Autodesk Inventor part; units mm, degrees
(part 4 of 6)
sketch "S09_267p4" plane through (0, 0, 0) normal (0, 0, 1) x (1, 0, 0)
  spline S0 degree 4 poles (184.2102, -33.211) (184.1723, -33.1957) (183.9876, -33.1195) (183.6772, -32.9928) (183.1534, -32.7788) (182.6023, -32.5533) (181.925, -32.2782) (181.1275, -31.9535) (180.2077, -31.5815) (179.1682, -31.1613) (178.009, -30.6956) (176.7313, -30.1834) (175.3365, -29.6271) (173.8252, -29.0272) (172.1997, -28.3847) (170.46, -27.7017) (168.6088, -26.9787) (166.6473, -26.2177) (164.5772, -25.419) (162.4002, -24.5854) (160.1184, -23.7178) (157.7339, -22.8179) (155.2484, -21.8869) (152.665, -20.9269) (149.9848, -19.9394) (147.2115, -18.9267) (144.3465, -17.889) (141.3934, -16.8298) (138.3539, -15.7493) (135.2318, -14.6509) (132.029, -13.5347) (128.7493, -12.404) (125.3952, -11.2596) (121.9703, -10.104) (118.4772, -8.9384) (114.92, -7.765) (111.3009, -6.5858) (107.6244, -5.4023) (103.8935, -4.2167) (100.1117, -3.0305) (96.2827, -1.8459) (92.4099, -0.6646) (88.4973, 0.5118) (84.5488, 1.6811) (80.5675, 2.8412) (76.5582, 3.9907) (72.5236, 5.1283) (68.4687, 6.2504) (64.3965, 7.3573) (60.3118, 8.4456) (56.2177, 9.5148) (52.1191, 10.5622) (48.0189, 11.5858) (43.9221, 12.5858) (39.832, 13.5582) (35.7496, 14.504) (31.6853, 15.4187) (27.6208, 16.3072) (23.5666, 17.1536) (19.5384, 17.959) (15.537, 18.7209) (11.5694, 19.4378) (7.6397, 20.1105) (3.7522, 20.7356) (-0.0895, 21.3157) (-3.8804, 21.8471) (-7.6174, 22.3317) (-11.2958, 22.7677) (-14.9121, 23.1565) (-18.462, 23.4964) (-21.9422, 23.7889) (-25.3485, 24.0333) (-28.6772, 24.2307) (-31.9251, 24.3805) (-35.0882, 24.4845) (-38.1632, 24.5425) (-41.1473, 24.5559) (-44.0366, 24.5247) (-46.8284, 24.4513) (-49.5195, 24.3353) (-52.1073, 24.178) (-54.5888, 23.9818) (-56.9615, 23.7464) (-59.2228, 23.4736) (-61.3709, 23.1653) (-63.4029, 22.8217) (-65.3171, 22.445) (-67.1116, 22.0362) (-68.7849, 21.5965) (-70.3349, 21.1268) (-71.761, 20.629) (-73.0614, 20.104) (-74.2351, 19.5519) (-75.2824, 18.9753) (-76.201, 18.3724) (-76.9918, 17.7451) (-77.6536, 17.0931) (-78.1852, 16.4152) (-78.5837, 15.7115) (-78.8483, 14.9847) (-78.9751, 14.2355) (-78.9672, 13.4757) (-78.8207, 12.7166) (-78.5387, 11.9594) (-78.1238, 11.2064) (-77.5783, 10.4572) (-76.904, 9.7121) (-76.102, 8.9696) (-75.1736, 8.2296) (-74.1195, 7.4923) (-72.9408, 6.7577) (-71.6387, 6.0264) (-70.2144, 5.2983) (-68.6696, 4.5743) (-67.0057, 3.8541) (-65.2248, 3.1392) (-63.3284, 2.4284) (-61.3186, 1.7241) (-59.1974, 1.0249) (-56.9673, 0.3318) (-54.63, -0.3546) (-52.1885, -1.0338) (-49.6448, -1.7073) (-47.0016, -2.3723) (-44.2618, -3.0312) (-41.4273, -3.6822) (-38.5019, -4.3262) (-35.488, -4.9635) (-32.3885, -5.5926) (-29.2065, -6.2163) (-25.9449, -6.8317) (-22.6074, -7.4421) (-19.1967, -8.0454) (-15.716, -8.6434) (-12.1695, -9.2365) (-8.5591, -9.8239) (-4.89, -10.4076) (-1.1645, -10.9871) (2.6133, -11.5629) (6.44, -12.1363) (10.3116, -12.7077) (14.2249, -13.2764) (18.1779, -13.8455) (22.1649, -14.4118) (26.1914, -14.983) (30.265, -15.5476) (34.3574, -16.1047) (38.4734, -16.6535) (42.6033, -17.1948) (46.7445, -17.7289) (50.8923, -18.2558) (55.0422, -18.7753) (59.1903, -19.2884) (63.3327, -19.7938) (67.465, -20.2937) (71.5831, -20.7858) (75.6829, -21.2723) (79.7601, -21.7518) (83.8113, -22.224) (87.8314, -22.6905) (91.817, -23.1497) (95.7643, -23.6014) (99.6691, -24.0469) (103.527, -24.4841) (107.3352, -24.9145) (111.0889, -25.3368) (114.7848, -25.7508) (118.4191, -26.1563) (121.9885, -26.5536) (125.4884, -26.9419) (128.9164, -27.3206) (132.2686, -27.6896) (135.5413, -28.0495) (138.7315, -28.398) (141.8361, -28.7371) (144.8517, -29.0645) (147.7753, -29.3818) (150.604, -29.6867) (153.3349, -29.9808) (155.9649, -30.2626) (158.4918, -30.5326) (160.9125, -30.7897) (163.2249, -31.0354) (165.4264, -31.2674) (167.5147, -31.4874) (169.4878, -31.6945) (171.3435, -31.8878) (173.0798, -32.0687) (174.6952, -32.2366) (176.1875, -32.3905) (177.5553, -32.5317) (178.7975, -32.659) (179.912, -32.7736) (180.8985, -32.8742) (181.755, -32.9616) (182.4819, -33.0358) (183.0744, -33.0955) (183.6373, -33.1534) (183.9708, -33.1866) (184.1695, -33.2068) (184.2102, -33.211) knots 0 0 0 0 0 0.003306 0.005253 0.00752 0.010062 0.01285 0.015861 0.019079 0.022488 0.026078 0.029837 0.033757 0.037828 0.042045 0.046398 0.050884 0.055494 0.060224 0.065069 0.070023 0.075082 0.080241 0.085495 0.090841 0.096274 0.101791 0.107386 0.113057 0.118799 0.124609 0.130484 0.136419 0.142412 0.148458 0.154554 0.160697 0.166884 0.17311 0.179374 0.185671 0.191998 0.198352 0.20473 0.211128 0.217543 0.223972 0.230412 0.23686 0.243312 0.249765 0.256217 0.262663 0.2691 0.275526 0.281941 0.288345 0.294734 0.301105 0.307451 0.313767 0.320049 0.326294 0.332498 0.338659 0.344773 0.350837 0.356848 0.362801 0.368695 0.374525 0.380288 0.38598 0.391599 0.39714 0.4026 0.407976 0.413263 0.418458 0.423557 0.428556 0.433452 0.438241 0.442917 0.447478 0.451919 0.456236 0.460425 0.464482 0.468403 0.472185 0.475825 0.479322 0.482675 0.485889 0.48897 0.49193 0.494788 0.497572 0.50031 0.503032 0.505769 0.508552 0.511409 0.514365 0.517441 0.520647 0.523991 0.527474 0.531098 0.534861 0.538758 0.542789 0.546947 0.551231 0.555634 0.560154 0.564786 0.569527 0.574371 0.579315 0.584356 0.58949 0.594712 0.60002 0.605409 0.610877 0.61642 0.622034 0.627716 0.633463 0.639271 0.645138 0.651061 0.657035 0.663059 0.669128 0.675241 0.681393 0.687582 0.693804 0.700057 0.706341 0.712655 0.718998 0.725365 0.731751 0.738149 0.744556 0.750969 0.757385 0.7638 0.770211 0.776616 0.783011 0.789393 0.795759 0.802106 0.808429 0.814727 0.820996 0.827232 0.833433 0.839595 0.845714 0.851788 0.857813 0.863785 0.869702 0.875558 0.881352 0.887078 0.892735 0.898316 0.90382 0.909242 0.914577 0.919822 0.924972 0.930023 0.93497 0.939808 0.944533 0.949139 0.95362 0.95797 0.962183 0.966252 0.970169 0.973927 0.977515 0.980924 0.984141 0.987151 0.989939 0.99248 0.994747 0.996694 1 1 1 1 1
  circle A0 centre (0, 0) radius 5.15
  line L0 (-32.24, 4.9) -> (-22.04, 4.9)
  line L1 (-22.04, 4.9) -> (-22.04, 9.1)
  line L2 (-22.04, 9.1) -> (-32.24, 9.1)
  line L3 (-32.24, 9.1) -> (-32.24, 4.9)
  line L4 (-32.24, 4.9) -> (-22.04, 9.1) construction
  line L5 (-22.04, 4.9) -> (-32.24, 9.1) construction
  line L6 (-58.58, 15.1) -> (-48.38, 15.1)
  line L7 (-48.38, 15.1) -> (-48.38, 10.9)
  line L8 (-48.38, 10.9) -> (-58.58, 10.9)
  line L9 (-58.58, 10.9) -> (-58.58, 15.1)
  line L10 (-58.58, 15.1) -> (-48.38, 10.9) construction
  line L11 (-48.38, 15.1) -> (-58.58, 10.9) construction
  line L12 (44.9, -2.9) -> (55.1, -2.9)
  line L13 (55.1, -2.9) -> (55.1, -7.1)
  line L14 (55.1, -7.1) -> (44.9, -7.1)
  line L15 (44.9, -7.1) -> (44.9, -2.9)
  line L16 (44.9, -2.9) -> (55.1, -7.1) construction
  line L17 (55.1, -2.9) -> (44.9, -7.1) construction
  line L18 (97.6, -12.9) -> (87.4, -12.9)
  line L19 (87.4, -12.9) -> (87.4, -17.1)
  line L20 (87.4, -17.1) -> (97.6, -17.1)
  line L21 (97.6, -17.1) -> (97.6, -12.9)
  line L22 (97.6, -12.9) -> (87.4, -17.1) construction
  line L23 (87.4, -12.9) -> (97.6, -17.1) construction
  point P0 (183.963, -33.1097)
  point P1 (183.654, -32.9833)
  point P2 (183.222, -32.8068)
  point P3 (182.6673, -32.5802)
  point P4 (181.9901, -32.3046)
  point P5 (181.1912, -31.9798)
  point P6 (180.2709, -31.6072)
  point P7 (179.2305, -31.187)
  point P8 (178.0707, -30.7206)
  point P9 (176.7923, -30.2083)
  point P10 (175.3966, -29.6516)
  point P11 (173.8846, -29.0513)
  point P12 (172.258, -28.4086)
  point P13 (170.5176, -27.7251)
  point P14 (168.6653, -27.0018)
  point P15 (166.7028, -26.2401)
  point P16 (164.6316, -25.4412)
  point P17 (162.4535, -24.607)
  point P18 (160.1705, -23.7389)
  point P19 (157.7848, -22.8384)
  point P20 (155.2981, -21.907)
  point P21 (152.7131, -20.9465)
  point P22 (150.0318, -19.9585)
  point P23 (147.2569, -18.9449)
  point P24 (144.3905, -17.907)
  point P25 (141.4358, -16.8469)
  point P26 (138.3948, -15.7661)
  point P27 (135.2711, -14.6669)
  point P28 (132.0668, -13.5503)
  point P29 (128.7852, -12.4188)
  point P30 (125.4295, -11.2739)
  point P31 (122.0028, -10.1176)
  point P32 (118.508, -8.9515)
  point P33 (114.9488, -7.7775)
  point P34 (111.328, -6.5976)
  point P35 (107.6495, -5.4135)
  point P36 (103.9167, -4.2273)
  point P37 (100.133, -3.0405)
  point P38 (96.302, -1.8553)
  point P39 (92.4272, -0.6734)
  point P40 (88.5126, 0.5035)
  point P41 (84.562, 1.6733)
  point P42 (80.5788, 2.8341)
  point P43 (76.5673, 3.9842)
  point P44 (72.5307, 5.1219)
  point P45 (68.4735, 6.2449)
  point P46 (64.3994, 7.352)
  point P47 (60.3125, 8.4409)
  point P48 (56.2163, 9.5104)
  point P49 (52.1154, 10.5581)
  point P50 (48.0133, 11.5824)
  point P51 (43.9144, 12.5822)
  point P52 (39.8223, 13.5553)
  point P53 (35.7415, 14.5002)
  point P54 (31.6757, 15.4153)
  point P55 (27.6092, 16.3014)
  point P56 (23.5509, 17.1494)
  point P57 (19.518, 17.955)
  point P58 (15.5145, 18.717)
  point P59 (11.5448, 19.4343)
  point P60 (7.6131, 20.1065)
  point P61 (3.7236, 20.7322)
  point P62 (-0.1199, 21.3115)
  point P63 (-3.9127, 21.8432)
  point P64 (-7.6514, 22.3273)
  point P65 (-11.3316, 22.7634)
  point P66 (-14.9496, 23.1516)
  point P67 (-18.5013, 23.4914)
  point P68 (-21.9831, 23.7833)
  point P69 (-25.3909, 24.0273)
  point P70 (-28.7211, 24.224)
  point P71 (-31.9705, 24.3734)
  point P72 (-35.135, 24.4766)
  point P73 (-38.2113, 24.534)
  point P74 (-41.1965, 24.5464)
  point P75 (-44.087, 24.5146)
  point P76 (-46.8798, 24.4399)
  point P77 (-49.5718, 24.3229)
  point P78 (-52.1604, 24.1646)
  point P79 (-54.6425, 23.9668)
  point P80 (-57.0157, 23.7301)
  point P81 (-59.2774, 23.4558)
  point P82 (-61.4255, 23.1456)
  point P83 (-63.4574, 22.8003)
  point P84 (-65.3711, 22.4215)
  point P85 (-67.1649, 22.0105)
  point P86 (-68.8368, 21.5683)
  point P87 (-70.3851, 21.0961)
  point P88 (-71.8087, 20.5955)
  point P89 (-73.1057, 20.0675)
  point P90 (-74.2751, 19.5129)
  point P91 (-75.3162, 18.9333)
  point P92 (-76.2275, 18.3289)
  point P93 (-77.0088, 17.7011)
  point P94 (-77.6594, 17.0508)
  point P95 (-78.1787, 16.3782)
  point P96 (-78.5664, 15.684)
  point P97 (-78.8227, 14.9689)
  point P98 (-78.9472, 14.2333)
  point P99 (-78.9396, 13.4872)
  point P100 (-78.7992, 12.7407)
  point P101 (-78.5268, 11.9944)
  point P102 (-78.1227, 11.2483)
  point P103 (-77.5877, 10.5027)
  point P104 (-76.9225, 9.7584)
  point P105 (-76.128, 9.0152)
  point P106 (-75.2056, 8.2737)
  point P107 (-74.1561, 7.5343)
  point P108 (-72.981, 6.7974)
  point P109 (-71.6816, 6.0638)
  point P110 (-70.2593, 5.3335)
  point P111 (-68.716, 4.6072)
  point P112 (-67.0531, 3.8852)
  point P113 (-65.2728, 3.168)
  point P114 (-63.3767, 2.4558)
  point P115 (-61.3671, 1.7495)
  point P116 (-59.2458, 1.0489)
  point P117 (-57.0153, 0.3544)
  point P118 (-54.6775, -0.3333)
  point P119 (-52.2353, -1.0141)
  point P120 (-49.6909, -1.6883)
  point P121 (-47.0469, -2.3549)
  point P122 (-44.3061, -3.0145)
  point P123 (-41.4707, -3.6667)
  point P124 (-38.5441, -4.3117)
  point P125 (-35.529, -4.9496)
  point P126 (-32.4283, -5.5801)
  point P127 (-29.245, -6.204)
  point P128 (-25.982, -6.8208)
  point P129 (-22.643, -7.4315)
  point P130 (-19.2309, -8.0358)
  point P131 (-15.7487, -8.6345)
  point P132 (-12.2004, -9.228)
  point P133 (-8.5887, -9.8164)
  point P134 (-4.9177, -10.4005)
  point P135 (-1.1906, -10.9807)
  point P136 (2.589, -11.5572)
  point P137 (6.4174, -12.1311)
  point P138 (10.2909, -12.7028)
  point P139 (14.2057, -13.2725)
  point P140 (18.1582, -13.8411)
  point P141 (22.1445, -14.4087)
  point P142 (26.1741, -14.9779)
  point P143 (30.25, -15.5434)
  point P144 (34.3485, -16.1011)
  point P145 (38.4663, -16.6506)
  point P146 (42.5987, -17.1924)
  point P147 (46.7418, -17.7269)
  point P148 (50.8917, -18.2542)
  point P149 (55.0437, -18.7742)
  point P150 (59.1939, -19.2874)
  point P151 (63.3384, -19.7936)
  point P152 (67.4728, -20.2934)
  point P153 (71.5931, -20.7862)
  point P154 (75.6949, -21.2728)
  point P155 (79.7742, -21.7526)
  point P156 (83.8274, -22.2254)
  point P157 (87.8497, -22.6919)
  point P158 (91.8373, -23.1514)
  point P159 (95.7866, -23.6037)
  point P160 (99.6934, -24.0491)
  point P161 (103.5535, -24.4869)
  point P162 (107.3635, -24.9173)
  point P163 (111.1193, -25.3398)
  point P164 (114.817, -25.754)
  point P165 (118.4533, -26.1599)
  point P166 (122.0244, -26.5573)
  point P167 (125.5263, -26.9458)
  point P168 (128.956, -27.3247)
  point P169 (132.31, -27.6941)
  point P170 (135.5845, -28.0538)
  point P171 (138.7764, -28.4029)
  point P172 (141.8826, -28.7417)
  point P173 (144.8998, -29.0697)
  point P174 (147.8249, -29.3868)
  point P175 (150.6552, -29.6922)
  point P176 (153.3875, -29.9861)
  point P177 (156.019, -30.2682)
  point P178 (158.5472, -30.5382)
  point P179 (160.9692, -30.7958)
  point P180 (163.2829, -31.0412)
  point P181 (165.4856, -31.2736)
  point P182 (167.5751, -31.4936)
  point P183 (169.5492, -31.7006)
  point P184 (171.406, -31.8943)
  point P185 (173.1433, -32.0752)
  point P186 (174.7596, -32.243)
  point P187 (176.2528, -32.3973)
  point P188 (177.6215, -32.5383)
  point P189 (178.8644, -32.666)
  point P190 (179.9798, -32.7804)
  point P191 (180.967, -32.8812)
  point P192 (181.8247, -32.9687)
  point P193 (182.5518, -33.0427)
  point P194 (183.1482, -33.1032)
  point P195 (183.6124, -33.1505)
  point P196 (183.9444, -33.184)
  point P197 (184.1437, -33.2042)
  point P198 (-27.14, 7)
  point P199 (-53.48, 13)
  dimension "d16" = 10.3
  dimension "d17" = 80.22
  dimension "d88" = 10.2
  dimension "d89" = 4.2
  dimension "d91" = 10.2
  dimension "d92" = 4.2
  dimension "d155" = 27.14
  dimension "d156" = 7
  dimension "d157" = 53.48
  dimension "d158" = 13
  dimension "d251" = 10.2
  dimension "d252" = 4.2
  dimension "d253" = 50
  dimension "d254" = 5
  dimension "d255" = 10.2
  dimension "d256" = 4.2
  dimension "d257" = 92.5
  dimension "d258" = 15
  constraints: 48 end point, 8 midpoint, 8 parallel, 4 horizontal, 4 perpendicular, 1 centre point, 201 other
  measures "d16" diameter of A0
  measures "d17" distance of A0.centre point (-78.947, 14.233)
  measures "d88" distance of L2.end L1.end
  measures "d89" distance of L1.end L0.end
  measures "d91" distance of L7.end L8.end
  measures "d92" distance of L6.end L7.end
  measures "d155" horizontal distance of point (-27.14, 7) point (0, 0)
  measures "d156" vertical distance of point (0, 0) point (-27.14, 7)
  measures "d157" horizontal distance of point (0, 0) point (-53.48, 13)
  measures "d158" vertical distance of point (0, 0) point (-53.48, 13)
  measures "d251" distance of L13.end L14.end
  measures "d252" distance of L12.end L13.end
  measures "d253" horizontal distance of point (50, -5) point (0, 0)
  measures "d254" vertical distance of point (0, 0) point (50, -5)
  measures "d255" distance of L20.end L19.end
  measures "d256" distance of L19.end L18.end
  measures "d257" horizontal distance of point (92.5, -15) point (0, 0)
  measures "d258" vertical distance of point (0, 0) point (92.5, -15)
sketch "S10_259p0" plane through (0, 0, 0) normal (0, 0, 1) x (1, 0, 0)
  spline S0 degree 4 poles (176.9199, -39.6111) (176.8839, -39.5948) (176.7082, -39.5135) (176.413, -39.3784) (175.9147, -39.15) (175.3906, -38.9094) (174.7463, -38.6158) (173.9877, -38.2692) (173.1127, -37.8719) (172.1237, -37.4231) (171.0208, -36.9253) (169.8051, -36.3778) (168.4779, -35.7829) (167.0397, -35.1411) (165.4927, -34.4534) (163.8368, -33.7219) (162.0747, -32.9471) (160.2073, -32.1311) (158.2364, -31.2742) (156.1634, -30.3792) (153.9905, -29.447) (151.7194, -28.4794) (149.3519, -27.4777) (146.8907, -26.4439) (144.3371, -25.3795) (141.6943, -24.2869) (138.9638, -23.1666) (136.149, -22.0217) (133.2513, -20.8528) (130.2746, -19.6633) (127.2204, -18.4532) (124.0923, -17.226) (120.8929, -15.9824) (117.6253, -14.7252) (114.2922, -13.4555) (110.8974, -12.1757) (107.4428, -10.8877) (103.9329, -9.5932) (100.3705, -8.2946) (96.7588, -6.9933) (93.1014, -5.6916) (89.4015, -4.3913) (85.6629, -3.0942) (81.8892, -1.8024) (78.0833, -0.5183) (74.25, 0.7568) (70.3918, 2.0213) (66.5132, 3.2717) (62.6173, 4.508) (58.7085, 5.7269) (54.7898, 6.9276) (50.8659, 8.1075) (46.9396, 9.2643) (43.0155, 10.3982) (39.0968, 11.5052) (35.1845, 12.5861) (31.2884, 13.636) (27.3911, 14.6608) (23.502, 15.6444) (19.6365, 16.5871) (15.7951, 17.4867) (11.9846, 18.3415) (8.2089, 19.1518) (4.4721, 19.9145) (0.7779, 20.6316) (-2.8691, 21.2996) (-6.4659, 21.9202) (-10.0079, 22.4913) (-13.4917, 23.0143) (-16.9134, 23.4872) (-20.2694, 23.9114) (-23.5559, 24.286) (-26.7691, 24.6121) (-29.9062, 24.8888) (-32.9631, 25.1177) (-35.9365, 25.2986) (-38.8238, 25.4326) (-41.6211, 25.5196) (-44.3259, 25.5618) (-46.9348, 25.5587) (-49.4455, 25.5114) (-51.8549, 25.4222) (-54.1606, 25.2906) (-56.36, 25.1183) (-58.4513, 24.9071) (-60.4316, 24.6571) (-62.2994, 24.3701) (-64.0526, 24.0473) (-65.6897, 23.6896) (-67.2087, 23.298) (-68.609, 22.8741) (-69.8888, 22.4188) (-71.047, 21.932) (-72.0839, 21.4165) (-72.9974, 20.8704) (-73.7881, 20.2954) (-74.4549, 19.6912) (-74.9969, 19.0568) (-75.4111, 18.3919) (-75.6966, 17.6993) (-75.8498, 16.9795) (-75.8728, 16.2439) (-75.7619, 15.5033) (-75.5197, 14.7591) (-75.1488, 14.0135) (-74.6512, 13.2664) (-74.0289, 12.518) (-73.2829, 11.7669) (-72.4145, 11.0132) (-71.4243, 10.2569) (-70.3134, 9.4982) (-69.083, 8.7377) (-67.7341, 7.9753) (-66.2686, 7.212) (-64.6876, 6.4475) (-62.9932, 5.6834) (-61.1867, 4.9187) (-59.2704, 4.1556) (-57.246, 3.3929) (-55.1159, 2.6317) (-52.8819, 1.8726) (-50.5466, 1.1164) (-48.1123, 0.3613) (-45.5814, -0.3893) (-42.9567, -1.1382) (-40.2401, -1.8831) (-37.4352, -2.625) (-34.5443, -3.3639) (-31.5704, -4.0985) (-28.5164, -4.8311) (-25.385, -5.5589) (-22.1799, -6.285) (-18.9037, -7.0072) (-15.5595, -7.7271) (-12.1515, -8.4449) (-8.6814, -9.1598) (-5.1544, -9.8735) (-1.5726, -10.5854) (2.06, -11.2959) (5.74, -12.0059) (9.4635, -12.716) (13.2274, -13.4251) (17.0299, -14.1361) (20.8652, -14.8459) (24.7387, -15.562) (28.658, -16.2736) (32.5957, -16.9787) (36.5567, -17.6767) (40.5314, -18.3681) (44.5173, -19.0529) (48.5099, -19.7311) (52.5048, -20.4021) (56.4983, -21.0669) (60.4865, -21.724) (64.4652, -22.3753) (68.4305, -23.0186) (72.3783, -23.6556) (76.3045, -24.2851) (80.2058, -24.9064) (84.0773, -25.5209) (87.9158, -26.1269) (91.7173, -26.7241) (95.4781, -27.3137) (99.1938, -27.8933) (102.8617, -28.4642) (106.4772, -29.0251) (110.037, -29.5757) (113.5376, -30.1156) (116.9757, -30.6447) (120.347, -31.1625) (123.649, -31.668) (126.8781, -32.1611) (130.0306, -32.6421) (133.1038, -33.1088) (136.0945, -33.5628) (138.9995, -34.002) (141.8158, -34.4277) (144.5409, -34.8374) (147.1718, -35.2328) (149.7055, -35.6122) (152.14, -35.9759) (154.4721, -36.323) (156.7, -36.6546) (158.821, -36.9684) (160.833, -37.2659) (162.734, -37.5463) (164.5221, -37.8087) (166.1949, -38.0542) (167.7514, -38.2822) (169.1894, -38.4917) (170.5073, -38.6838) (171.7043, -38.8574) (172.7781, -39.0135) (173.7288, -39.1508) (174.5541, -39.2702) (175.2545, -39.3715) (175.8255, -39.4533) (176.3679, -39.5321) (176.6893, -39.5777) (176.8807, -39.6054) (176.9199, -39.6111) knots 0 0 0 0 0 0.003306 0.005253 0.00752 0.010062 0.01285 0.015861 0.019079 0.022488 0.026078 0.029837 0.033757 0.037828 0.042045 0.046398 0.050884 0.055494 0.060224 0.065069 0.070023 0.075082 0.080241 0.085495 0.090841 0.096274 0.101791 0.107386 0.113057 0.118799 0.124609 0.130484 0.136419 0.142412 0.148458 0.154554 0.160697 0.166884 0.17311 0.179374 0.185671 0.191998 0.198352 0.20473 0.211128 0.217543 0.223972 0.230412 0.23686 0.243312 0.249765 0.256217 0.262663 0.2691 0.275526 0.281941 0.288345 0.294734 0.301105 0.307451 0.313767 0.320049 0.326294 0.332498 0.338659 0.344773 0.350837 0.356848 0.362801 0.368695 0.374525 0.380288 0.38598 0.391599 0.39714 0.4026 0.407976 0.413263 0.418458 0.423557 0.428556 0.433452 0.438241 0.442917 0.447478 0.451919 0.456236 0.460425 0.464482 0.468403 0.472185 0.475825 0.479322 0.482675 0.485889 0.48897 0.49193 0.494788 0.497572 0.50031 0.503032 0.505769 0.508552 0.511409 0.514365 0.517441 0.520647 0.523991 0.527474 0.531098 0.534861 0.538758 0.542789 0.546947 0.551231 0.555634 0.560154 0.564786 0.569527 0.574371 0.579315 0.584356 0.58949 0.594712 0.60002 0.605409 0.610877 0.61642 0.622034 0.627716 0.633463 0.639271 0.645138 0.651061 0.657035 0.663059 0.669128 0.675241 0.681393 0.687582 0.693804 0.700057 0.706341 0.712655 0.718998 0.725365 0.731751 0.738149 0.744556 0.750969 0.757385 0.7638 0.770211 0.776616 0.783011 0.789393 0.795759 0.802106 0.808429 0.814727 0.820996 0.827232 0.833433 0.839595 0.845714 0.851788 0.857813 0.863785 0.869702 0.875558 0.881352 0.887078 0.892735 0.898316 0.90382 0.909242 0.914577 0.919822 0.924972 0.930023 0.93497 0.939808 0.944533 0.949139 0.95362 0.95797 0.962183 0.966252 0.970169 0.973927 0.977515 0.980924 0.984141 0.987151 0.989939 0.99248 0.994747 0.996694 1 1 1 1 1
  circle A0 centre (0, 0) radius 5.15
  line L0 (-48.38, 15.1) -> (-58.58, 15.1)
  line L1 (-58.58, 15.1) -> (-58.58, 10.9)
  line L2 (-58.58, 10.9) -> (-48.38, 10.9)
  line L3 (-48.38, 10.9) -> (-48.38, 15.1)
  line L4 (-48.38, 15.1) -> (-58.58, 10.9) construction
  line L5 (-58.58, 15.1) -> (-48.38, 10.9) construction
  line L6 (-31, 10.1) -> (-20.8, 10.1)
  line L7 (-20.8, 10.1) -> (-20.8, 5.9)
  line L8 (-20.8, 5.9) -> (-31, 5.9)
  line L9 (-31, 5.9) -> (-31, 10.1)
  line L10 (-31, 10.1) -> (-20.8, 5.9) construction
  line L11 (-20.8, 10.1) -> (-31, 5.9) construction
  line L12 (87.4, -12.9) -> (97.6, -12.9)
  line L13 (97.6, -12.9) -> (97.6, -17.1)
  line L14 (97.6, -17.1) -> (87.4, -17.1)
  line L15 (87.4, -17.1) -> (87.4, -12.9)
  line L16 (87.4, -12.9) -> (97.6, -17.1) construction
  line L17 (97.6, -12.9) -> (87.4, -17.1) construction
  line L18 (49.35, -4.9) -> (39.15, -4.9)
  line L19 (39.15, -4.9) -> (39.15, -9.1)
  line L20 (39.15, -9.1) -> (49.35, -9.1)
  line L21 (49.35, -9.1) -> (49.35, -4.9)
  line L22 (49.35, -4.9) -> (39.15, -9.1) construction
  line L23 (39.15, -4.9) -> (49.35, -9.1) construction
  point P0 (0, 0)
  point P1 (176.6848, -39.503)
  point P2 (176.3909, -39.3682)
  point P3 (175.98, -39.1799)
  point P4 (175.4524, -38.9381)
  point P5 (174.8083, -38.6439)
  point P6 (174.0482, -38.2972)
  point P7 (173.1728, -37.8992)
  point P8 (172.183, -37.4504)
  point P9 (171.0795, -36.952)
  point P10 (169.8631, -36.4045)
  point P11 (168.5351, -35.8091)
  point P12 (167.0962, -35.1668)
  point P13 (165.5481, -34.4789)
  point P14 (163.8916, -33.7468)
  point P15 (162.1284, -32.9717)
  point P16 (160.2602, -32.155)
  point P17 (158.2882, -31.2979)
  point P18 (156.2141, -30.4022)
  point P19 (154.0401, -29.4695)
  point P20 (151.7678, -28.5014)
  point P21 (149.3991, -27.4991)
  point P22 (146.9365, -26.4647)
  point P23 (144.3817, -25.3999)
  point P24 (141.7375, -24.3065)
  point P25 (139.0057, -23.1858)
  point P26 (136.1893, -22.04)
  point P27 (133.2903, -20.8708)
  point P28 (130.3119, -19.6803)
  point P29 (127.2563, -18.4698)
  point P30 (124.1265, -17.2417)
  point P31 (120.9255, -15.9977)
  point P32 (117.6562, -14.7396)
  point P33 (114.3215, -13.4694)
  point P34 (110.9247, -12.1889)
  point P35 (107.4686, -10.9002)
  point P36 (103.9568, -9.6051)
  point P37 (100.3926, -8.3058)
  point P38 (96.7791, -7.0039)
  point P39 (93.1197, -5.7015)
  point P40 (89.4179, -4.4005)
  point P41 (85.6773, -3.1028)
  point P42 (81.9016, -1.8105)
  point P43 (78.094, -0.5257)
  point P44 (74.2585, 0.75)
  point P45 (70.3984, 2.0148)
  point P46 (66.5177, 3.2661)
  point P47 (62.6199, 4.5027)
  point P48 (58.709, 5.7223)
  point P49 (54.7883, 6.9234)
  point P50 (50.8623, 8.1036)
  point P51 (46.934, 9.2613)
  point P52 (43.0079, 10.3951)
  point P53 (39.0873, 11.5028)
  point P54 (35.1765, 12.5827)
  point P55 (31.279, 13.6332)
  point P56 (27.3797, 14.6556)
  point P57 (23.4866, 15.6409)
  point P58 (19.6166, 16.584)
  point P59 (15.7731, 17.4838)
  point P60 (11.9606, 18.339)
  point P61 (8.183, 19.149)
  point P62 (4.4444, 19.9122)
  point P63 (0.7484, 20.6288)
  point P64 (-2.9005, 21.2972)
  point P65 (-6.499, 21.9173)
  point P66 (-10.0428, 22.4886)
  point P67 (-13.5282, 23.011)
  point P68 (-16.9516, 23.4839)
  point P69 (-20.3092, 23.9076)
  point P70 (-23.5971, 24.282)
  point P71 (-26.812, 24.6073)
  point P72 (-29.9504, 24.8838)
  point P73 (-33.0086, 25.112)
  point P74 (-35.9833, 25.2923)
  point P75 (-38.8717, 25.4254)
  point P76 (-41.6703, 25.5119)
  point P77 (-44.376, 25.5529)
  point P78 (-46.9859, 25.5488)
  point P79 (-49.4974, 25.5006)
  point P80 (-51.9075, 25.4099)
  point P81 (-54.2137, 25.277)
  point P82 (-56.4135, 25.1034)
  point P83 (-58.5049, 24.8903)
  point P84 (-60.4852, 24.6386)
  point P85 (-62.3526, 24.3496)
  point P86 (-64.1052, 24.0246)
  point P87 (-65.7411, 23.6644)
  point P88 (-67.2586, 23.2703)
  point P89 (-68.6565, 22.8436)
  point P90 (-69.9331, 22.3852)
  point P91 (-71.0873, 21.896)
  point P92 (-72.1183, 21.3773)
  point P93 (-73.0247, 20.8294)
  point P94 (-73.8063, 20.2535)
  point P95 (-74.4623, 19.6506)
  point P96 (-74.9921, 19.0207)
  point P97 (-75.3954, 18.3647)
  point P98 (-75.6725, 17.683)
  point P99 (-75.8228, 16.9762)
  point P100 (-75.8457, 16.2538)
  point P101 (-75.7401, 15.5258)
  point P102 (-75.5067, 14.7925)
  point P103 (-75.146, 14.054)
  point P104 (-74.6585, 13.3108)
  point P105 (-74.0449, 12.5635)
  point P106 (-73.3062, 11.8121)
  point P107 (-72.4436, 11.0571)
  point P108 (-71.458, 10.299)
  point P109 (-70.3507, 9.5383)
  point P110 (-69.123, 8.7756)
  point P111 (-67.7762, 8.0111)
  point P112 (-66.3121, 7.2457)
  point P113 (-64.7322, 6.4795)
  point P114 (-63.0384, 5.7133)
  point P115 (-61.2324, 4.9472)
  point P116 (-59.3162, 4.1822)
  point P117 (-57.2918, 3.4181)
  point P118 (-55.1614, 2.6555)
  point P119 (-52.927, 1.8952)
  point P120 (-50.5912, 1.1373)
  point P121 (-48.1561, 0.3816)
  point P122 (-45.6245, -0.3707)
  point P123 (-42.9989, -1.1202)
  point P124 (-40.2814, -1.8664)
  point P125 (-37.4754, -2.6093)
  point P126 (-34.5835, -3.3488)
  point P127 (-31.6084, -4.0847)
  point P128 (-28.553, -4.8177)
  point P129 (-25.4204, -5.5469)
  point P130 (-22.2139, -6.2733)
  point P131 (-18.9364, -6.9965)
  point P132 (-15.5908, -7.7171)
  point P133 (-12.1811, -8.4355)
  point P134 (-8.7097, -9.1514)
  point P135 (-5.1809, -9.8655)
  point P136 (-1.5976, -10.5781)
  point P137 (2.0367, -11.2893)
  point P138 (5.7184, -12)
  point P139 (9.4436, -12.7104)
  point P140 (13.209, -13.4205)
  point P141 (17.0109, -14.131)
  point P142 (20.8457, -14.842)
  point P143 (24.7221, -15.5563)
  point P144 (28.6436, -16.2689)
  point P145 (32.5872, -16.9748)
  point P146 (36.5499, -17.6736)
  point P147 (40.527, -18.3655)
  point P148 (44.5148, -19.0508)
  point P149 (48.5094, -19.7294)
  point P150 (52.5063, -20.4011)
  point P151 (56.5018, -21.0661)
  point P152 (60.492, -21.724)
  point P153 (64.4728, -22.3754)
  point P154 (68.4401, -23.0194)
  point P155 (72.3899, -23.6566)
  point P156 (76.3182, -24.2864)
  point P157 (80.2214, -24.9084)
  point P158 (84.095, -25.523)
  point P159 (87.9353, -26.1294)
  point P160 (91.7389, -26.7272)
  point P161 (95.5015, -27.3167)
  point P162 (99.2193, -27.897)
  point P163 (102.889, -28.4681)
  point P164 (106.5064, -29.0293)
  point P165 (110.0681, -29.5801)
  point P166 (113.5705, -30.1204)
  point P167 (117.0104, -30.6498)
  point P168 (120.3835, -31.1678)
  point P169 (123.6872, -31.6736)
  point P170 (126.918, -32.1671)
  point P171 (130.0722, -32.648)
  point P172 (133.147, -33.1153)
  point P173 (136.1392, -33.5692)
  point P174 (139.0458, -34.009)
  point P175 (141.8637, -34.4345)
  point P176 (144.5902, -34.8448)
  point P177 (147.2225, -35.2401)
  point P178 (149.7576, -35.6198)
  point P179 (152.1933, -35.9836)
  point P180 (154.5268, -36.3311)
  point P181 (156.7558, -36.6625)
  point P182 (158.878, -36.9768)
  point P183 (160.8912, -37.2744)
  point P184 (162.7932, -37.5548)
  point P185 (164.5822, -37.8176)
  point P186 (166.2561, -38.0631)
  point P187 (167.8135, -38.291)
  point P188 (169.2523, -38.5009)
  point P189 (170.5711, -38.6929)
  point P190 (171.7687, -38.8668)
  point P191 (172.8435, -39.0228)
  point P192 (173.7947, -39.1604)
  point P193 (174.6213, -39.2799)
  point P194 (175.3219, -39.381)
  point P195 (175.8965, -39.4638)
  point P196 (176.3439, -39.5284)
  point P197 (176.6638, -39.5742)
  point P198 (176.8559, -39.6018)
  point P199 (-53.48, 13)
  dimension "d19" = 10.3
  dimension "d20" = 77.7
  dimension "d94" = 10.2
  dimension "d95" = 4.2
  dimension "d97" = 10.2
  dimension "d98" = 4.2
  dimension "d159" = 53.48
  dimension "d160" = 13
  dimension "d161" = 0
  dimension "d162" = 25.9
  dimension "d163" = 8
  dimension "d259" = 10.2
  dimension "d260" = 4.2
  dimension "d261" = 92.5
  dimension "d262" = 15
  dimension "d263" = 10.2
  dimension "d264" = 4.2
  dimension "d265" = 44.25
  dimension "d266" = 7
  constraints: 48 end point, 8 midpoint, 8 parallel, 4 horizontal, 4 perpendicular, 1 centre point, 201 other
  measures "d19" diameter of A0
  measures "d20" distance of A0.centre point (-75.823, 16.976)
  measures "d94" distance of L2.end L1.end
  measures "d95" distance of L1.end L0.end
  measures "d97" distance of L7.end L8.end
  measures "d98" distance of L6.end L7.end
  measures "d159" horizontal distance of point (0, 0) point (-53.48, 13)
  measures "d160" vertical distance of A0.centre point (-53.48, 13)
  measures "d161" distance of point (0, 0) A0.centre
  measures "d162" horizontal distance of A0.centre point (-25.9, 8)
  measures "d163" vertical distance of A0.centre point (-25.9, 8)
  measures "d259" distance of L13.end L14.end
  measures "d260" distance of L12.end L13.end
  measures "d261" horizontal distance of point (92.5, -15) point (0, 0)
  measures "d262" vertical distance of point (0, 0) point (92.5, -15)
  measures "d263" distance of L20.end L19.end
  measures "d264" distance of L19.end L18.end
  measures "d265" horizontal distance of point (44.25, -7) point (0, 0)
  measures "d266" vertical distance of point (0, 0) point (44.25, -7)
sketch "S11_257p6" plane through (0, 0, 0) normal (0, 0, 1) x (1, 0, 0)
  spline S0 degree 4 poles (174.4655, -45.575) (174.4303, -45.5574) (174.2586, -45.4705) (173.9698, -45.3258) (173.4826, -45.0814) (172.9701, -44.8239) (172.34, -44.5094) (171.598, -44.1383) (170.7422, -43.7127) (169.775, -43.2319) (168.6962, -42.6985) (167.507, -42.1117) (166.2086, -41.4738) (164.8016, -40.7855) (163.288, -40.0477) (161.6678, -39.2625) (159.9434, -38.4306) (158.1159, -37.5541) (156.1869, -36.6332) (154.1578, -35.6709) (152.0306, -34.6682) (149.8071, -33.6268) (147.4889, -32.5481) (145.0788, -31.4343) (142.5779, -30.2868) (139.9894, -29.1081) (137.3146, -27.8988) (134.5569, -26.6622) (131.7176, -25.3987) (128.8005, -24.112) (125.8072, -22.8021) (122.741, -21.4726) (119.6044, -20.1244) (116.4006, -18.7602) (113.132, -17.3813) (109.8025, -15.9902) (106.414, -14.5889) (102.9706, -13.1791) (99.4752, -11.7634) (95.9308, -10.3433) (92.3411, -8.9213) (88.709, -7.4991) (85.0384, -6.0787) (81.3328, -4.6624) (77.5948, -3.2526) (73.8293, -1.8508) (70.0386, -0.4587) (66.2272, 0.9202) (62.3982, 2.2856) (58.5557, 3.6342) (54.7027, 4.965) (50.8438, 6.2754) (46.9816, 7.5629) (43.121, 8.8276) (39.2647, 10.0652) (35.4138, 11.2768) (31.578, 12.457) (27.7401, 13.6122) (23.9089, 14.7262) (20.0997, 15.7987) (16.313, 16.8276) (12.5554, 17.8108) (8.8309, 18.7486) (5.1434, 19.6377) (1.4966, 20.4801) (-2.1051, 21.2719) (-5.6584, 22.0148) (-9.1591, 22.7067) (-12.6036, 23.3486) (-15.9881, 23.9386) (-19.309, 24.478) (-22.5626, 24.9655) (-25.7451, 25.4023) (-28.8535, 25.7873) (-31.884, 26.1221) (-34.8331, 26.406) (-37.6983, 26.6405) (-40.4757, 26.825) (-43.1627, 26.9618) (-45.7561, 27.0502) (-48.2533, 27.0912) (-50.6513, 27.087) (-52.9477, 27.037) (-55.14, 26.9429) (-57.226, 26.8063) (-59.2032, 26.6271) (-61.0698, 26.4074) (-62.8237, 26.148) (-64.4636, 25.8499) (-65.9871, 25.5138) (-67.3938, 25.1416) (-68.6819, 24.7339) (-69.8502, 24.2907) (-70.8989, 23.8146) (-71.826, 23.3038) (-72.6321, 22.76) (-73.3161, 22.1829) (-73.8771, 21.5713) (-74.3121, 20.9249) (-74.6202, 20.2465) (-74.7976, 19.5363) (-74.8464, 18.806) (-74.762, 18.066) (-74.5474, 17.3177) (-74.2048, 16.5637) (-73.7365, 15.8036) (-73.1441, 15.0379) (-72.4289, 14.2651) (-71.5922, 13.4855) (-70.6345, 12.6991) (-69.5569, 11.906) (-68.3605, 11.1069) (-67.0466, 10.3018) (-65.6166, 9.4917) (-64.0719, 8.6765) (-62.4145, 7.8576) (-60.6457, 7.0341) (-58.7677, 6.2084) (-56.7822, 5.3794) (-54.6917, 4.5481) (-52.4977, 3.7153) (-50.203, 2.8817) (-47.8098, 2.0459) (-45.3205, 1.211) (-42.7378, 0.3747) (-40.0637, -0.461) (-37.3017, -1.2968) (-34.4542, -2.1326) (-31.5239, -2.967) (-28.514, -3.8023) (-25.4269, -4.6355) (-22.2666, -5.4696) (-19.0355, -6.3022) (-15.7367, -7.1351) (-12.3743, -7.968) (-8.9503, -8.8003) (-5.4695, -9.6333) (-1.9342, -10.4665) (1.6516, -11.3) (5.2845, -12.1348) (8.9607, -12.9711) (12.6771, -13.8079) (16.4317, -14.6479) (20.2191, -15.4879) (24.0441, -16.3355) (27.9148, -17.1802) (31.8041, -18.0191) (35.7168, -18.8518) (39.6433, -19.6784) (43.5812, -20.4988) (47.5259, -21.3129) (51.4733, -22.1199) (55.4194, -22.9207) (59.3606, -23.7137) (63.2925, -24.5006) (67.2114, -25.2789) (71.113, -26.0506) (74.9935, -26.8139) (78.8495, -27.5682) (82.6762, -28.3148) (86.4702, -29.0517) (90.228, -29.7786) (93.9454, -30.4964) (97.6185, -31.2028) (101.2442, -31.8988) (104.8183, -32.5831) (108.3374, -33.2552) (111.7979, -33.9145) (115.1968, -34.5611) (118.5296, -35.1939) (121.794, -35.8122) (124.9863, -36.4155) (128.103, -37.0041) (131.1413, -37.5757) (134.0981, -38.1318) (136.9702, -38.6702) (139.7546, -39.1921) (142.449, -39.6949) (145.0501, -40.1801) (147.5552, -40.646) (149.9623, -41.0929) (152.2682, -41.5197) (154.471, -41.9273) (156.5683, -42.3136) (158.5578, -42.6799) (160.4375, -43.0253) (162.2056, -43.3488) (163.8598, -43.6514) (165.3989, -43.9326) (166.8208, -44.1912) (168.1241, -44.4284) (169.3078, -44.6429) (170.3697, -44.8357) (171.3098, -45.0055) (172.126, -45.1531) (172.8185, -45.2784) (173.3833, -45.3797) (173.9196, -45.4771) (174.2375, -45.5337) (174.4268, -45.5679) (174.4655, -45.575) knots 0 0 0 0 0 0.003306 0.005253 0.00752 0.010062 0.01285 0.015861 0.019079 0.022488 0.026078 0.029837 0.033757 0.037828 0.042045 0.046398 0.050884 0.055494 0.060224 0.065069 0.070023 0.075082 0.080241 0.085495 0.090841 0.096274 0.101791 0.107386 0.113057 0.118799 0.124609 0.130484 0.136419 0.142412 0.148458 0.154554 0.160697 0.166884 0.17311 0.179374 0.185671 0.191998 0.198352 0.20473 0.211128 0.217543 0.223972 0.230412 0.23686 0.243312 0.249765 0.256217 0.262663 0.2691 0.275526 0.281941 0.288345 0.294734 0.301105 0.307451 0.313767 0.320049 0.326294 0.332498 0.338659 0.344773 0.350837 0.356848 0.362801 0.368695 0.374525 0.380288 0.38598 0.391599 0.39714 0.4026 0.407976 0.413263 0.418458 0.423557 0.428556 0.433452 0.438241 0.442917 0.447478 0.451919 0.456236 0.460425 0.464482 0.468403 0.472185 0.475825 0.479322 0.482675 0.485889 0.48897 0.49193 0.494788 0.497572 0.50031 0.503032 0.505769 0.508552 0.511409 0.514365 0.517441 0.520647 0.523991 0.527474 0.531098 0.534861 0.538758 0.542789 0.546947 0.551231 0.555634 0.560154 0.564786 0.569527 0.574371 0.579315 0.584356 0.58949 0.594712 0.60002 0.605409 0.610877 0.61642 0.622034 0.627716 0.633463 0.639271 0.645138 0.651061 0.657035 0.663059 0.669128 0.675241 0.681393 0.687582 0.693804 0.700057 0.706341 0.712655 0.718998 0.725365 0.731751 0.738149 0.744556 0.750969 0.757385 0.7638 0.770211 0.776616 0.783011 0.789393 0.795759 0.802106 0.808429 0.814727 0.820996 0.827232 0.833433 0.839595 0.845714 0.851788 0.857813 0.863785 0.869702 0.875558 0.881352 0.887078 0.892735 0.898316 0.90382 0.909242 0.914577 0.919822 0.924972 0.930023 0.93497 0.939808 0.944533 0.949139 0.95362 0.95797 0.962183 0.966252 0.970169 0.973927 0.977515 0.980924 0.984141 0.987151 0.989939 0.99248 0.994747 0.996694 1 1 1 1 1
  circle A0 centre (0, 0) radius 5.15
  line L0 (-31, 5.9) -> (-20.8, 5.9)
  line L1 (-20.8, 5.9) -> (-20.8, 10.1)
  line L2 (-20.8, 10.1) -> (-31, 10.1)
  line L3 (-31, 10.1) -> (-31, 5.9)
  line L4 (-31, 5.9) -> (-20.8, 10.1) construction
  line L5 (-20.8, 5.9) -> (-31, 10.1) construction
  line L6 (-56.62, 15.9) -> (-46.42, 15.9)
  line L7 (-46.42, 15.9) -> (-46.42, 20.1)
  line L8 (-46.42, 20.1) -> (-56.62, 20.1)
  line L9 (-56.62, 20.1) -> (-56.62, 15.9)
  line L10 (-56.62, 15.9) -> (-46.42, 20.1) construction
  line L11 (-46.42, 15.9) -> (-56.62, 20.1) construction
  line L12 (49.35, -4.9) -> (39.15, -4.9)
  line L13 (39.15, -4.9) -> (39.15, -9.1)
  line L14 (39.15, -9.1) -> (49.35, -9.1)
  line L15 (49.35, -9.1) -> (49.35, -4.9)
  line L16 (49.35, -4.9) -> (39.15, -9.1) construction
  line L17 (39.15, -4.9) -> (49.35, -9.1) construction
  line L18 (75.1, -19.1) -> (64.9, -19.1)
  line L19 (64.9, -19.1) -> (64.9, -14.9)
  line L20 (64.9, -14.9) -> (75.1, -14.9)
  line L21 (75.1, -14.9) -> (75.1, -19.1)
  line L22 (75.1, -19.1) -> (64.9, -14.9) construction
  line L23 (64.9, -19.1) -> (75.1, -14.9) construction
  point P0 (174.2356, -45.4593)
  point P1 (173.9483, -45.315)
  point P2 (173.5464, -45.1133)
  point P3 (173.0305, -44.8545)
  point P4 (172.4005, -44.5395)
  point P5 (171.6572, -44.1683)
  point P6 (170.8011, -43.742)
  point P7 (169.8329, -43.2612)
  point P8 (168.7536, -42.7271)
  point P9 (167.5637, -42.1402)
  point P10 (166.2645, -41.5018)
  point P11 (164.8568, -40.813)
  point P12 (163.3422, -40.075)
  point P13 (161.7213, -39.2892)
  point P14 (159.9959, -38.4569)
  point P15 (158.1676, -37.5797)
  point P16 (156.2375, -36.6586)
  point P17 (154.2073, -35.6956)
  point P18 (152.0791, -34.6923)
  point P19 (149.8544, -33.6503)
  point P20 (147.5351, -32.5711)
  point P21 (145.1236, -31.4566)
  point P22 (142.6216, -30.3086)
  point P23 (140.0316, -29.1291)
  point P24 (137.3556, -27.9194)
  point P25 (134.5963, -26.6818)
  point P26 (131.7558, -25.4179)
  point P27 (128.837, -24.1302)
  point P28 (125.8422, -22.8199)
  point P29 (122.7744, -21.4895)
  point P30 (119.6363, -20.1407)
  point P31 (116.4308, -18.7756)
  point P32 (113.1606, -17.3961)
  point P33 (109.8293, -16.0043)
  point P34 (106.4391, -14.6022)
  point P35 (102.9939, -13.1918)
  point P36 (99.4967, -11.7753)
  point P37 (95.9506, -10.3545)
  point P38 (92.3589, -8.9317)
  point P39 (88.725, -7.5088)
  point P40 (85.0525, -6.0878)
  point P41 (81.3448, -4.6709)
  point P42 (77.6052, -3.2603)
  point P43 (73.8375, -1.8578)
  point P44 (70.045, -0.4653)
  point P45 (66.2315, 0.9145)
  point P46 (62.4005, 2.2803)
  point P47 (58.5559, 3.6296)
  point P48 (54.701, 4.9609)
  point P49 (50.84, 6.2717)
  point P50 (46.976, 7.5601)
  point P51 (43.1133, 8.8247)
  point P52 (39.2552, 10.0631)
  point P53 (35.4057, 11.2737)
  point P54 (31.5685, 12.4545)
  point P55 (27.7285, 13.6075)
  point P56 (23.8935, 14.7233)
  point P57 (20.0798, 15.7964)
  point P58 (16.2911, 16.8256)
  point P59 (12.5315, 17.8093)
  point P60 (8.8051, 18.7468)
  point P61 (5.1157, 19.6365)
  point P62 (1.4671, 20.4783)
  point P63 (-2.1364, 21.2706)
  point P64 (-5.6914, 22.0131)
  point P65 (-9.1939, 22.7052)
  point P66 (-12.64, 23.3466)
  point P67 (-16.0262, 23.9367)
  point P68 (-19.3487, 24.4756)
  point P69 (-22.6037, 24.963)
  point P70 (-25.7878, 25.3991)
  point P71 (-28.8976, 25.7839)
  point P72 (-31.9294, 26.1179)
  point P73 (-34.8799, 26.4014)
  point P74 (-37.7462, 26.635)
  point P75 (-40.5249, 26.8191)
  point P76 (-43.2129, 26.9547)
  point P77 (-45.8072, 27.0421)
  point P78 (-48.3052, 27.0823)
  point P79 (-50.704, 27.0766)
  point P80 (-53.001, 27.0254)
  point P81 (-55.1937, 26.9299)
  point P82 (-57.2799, 26.7914)
  point P83 (-59.2571, 26.6106)
  point P84 (-61.1234, 26.3889)
  point P85 (-62.8768, 26.1273)
  point P86 (-64.5155, 25.8266)
  point P87 (-66.0377, 25.4881)
  point P88 (-67.4421, 25.113)
  point P89 (-68.7271, 24.7021)
  point P90 (-69.8915, 24.2562)
  point P91 (-70.9345, 23.7768)
  point P92 (-71.8546, 23.264)
  point P93 (-72.6517, 22.719)
  point P94 (-73.3249, 22.1427)
  point P95 (-73.8736, 21.5352)
  point P96 (-74.2975, 20.8973)
  point P97 (-74.5968, 20.2294)
  point P98 (-74.7709, 19.5321)
  point P99 (-74.8191, 18.8149)
  point P100 (-74.7396, 18.0876)
  point P101 (-74.5333, 17.3505)
  point P102 (-74.2007, 16.6038)
  point P103 (-73.7421, 15.848)
  point P104 (-73.1585, 15.0837)
  point P105 (-72.4506, 14.3109)
  point P106 (-71.6196, 13.5302)
  point P107 (-70.6665, 12.7421)
  point P108 (-69.5925, 11.9471)
  point P109 (-68.3989, 11.146)
  point P110 (-67.0871, 10.339)
  point P111 (-65.6587, 9.5268)
  point P112 (-64.1151, 8.7098)
  point P113 (-62.4584, 7.8889)
  point P114 (-60.6901, 7.0641)
  point P115 (-58.8123, 6.2365)
  point P116 (-56.8268, 5.406)
  point P117 (-54.736, 4.5734)
  point P118 (-52.5417, 3.7393)
  point P119 (-50.2466, 2.9041)
  point P120 (-47.8527, 2.0676)
  point P121 (-45.3627, 1.231)
  point P122 (-42.7792, 0.394)
  point P123 (-40.1042, -0.4429)
  point P124 (-37.3412, -1.2797)
  point P125 (-34.4926, -2.1163)
  point P126 (-31.5612, -2.952)
  point P127 (-28.55, -3.7876)
  point P128 (-25.4618, -4.6223)
  point P129 (-22.3001, -5.4567)
  point P130 (-19.0676, -6.2905)
  point P131 (-15.7675, -7.1241)
  point P132 (-12.4034, -7.9576)
  point P133 (-8.9781, -8.7909)
  point P134 (-5.4956, -9.6245)
  point P135 (-1.9588, -10.4584)
  point P136 (1.6286, -11.2927)
  point P137 (5.2632, -12.1282)
  point P138 (8.9411, -12.9649)
  point P139 (12.659, -13.8027)
  point P140 (16.4131, -14.6423)
  point P141 (20.1998, -15.4834)
  point P142 (24.0279, -16.3293)
  point P143 (27.9007, -17.1751)
  point P144 (31.7958, -18.015)
  point P145 (35.7102, -18.8485)
  point P146 (39.639, -19.6757)
  point P147 (43.5788, -20.4966)
  point P148 (47.5255, -21.3112)
  point P149 (51.4748, -22.1189)
  point P150 (55.423, -22.92)
  point P151 (59.3661, -23.7139)
  point P152 (63.3001, -24.5009)
  point P153 (67.2209, -25.2801)
  point P154 (71.1245, -26.052)
  point P155 (75.007, -26.8157)
  point P156 (78.8649, -27.5708)
  point P157 (82.6936, -28.3175)
  point P158 (86.4896, -29.0548)
  point P159 (90.2493, -29.7824)
  point P160 (93.9686, -30.5003)
  point P161 (97.6437, -31.2074)
  point P162 (101.2712, -31.9036)
  point P163 (104.8472, -32.5883)
  point P164 (108.3681, -33.2607)
  point P165 (111.8305, -33.9205)
  point P166 (115.231, -34.5673)
  point P167 (118.5657, -35.2004)
  point P168 (121.8317, -35.819)
  point P169 (125.0258, -36.4228)
  point P170 (128.1442, -37.0114)
  point P171 (131.184, -37.5837)
  point P172 (134.1423, -38.1398)
  point P173 (137.016, -38.6788)
  point P174 (139.802, -39.2005)
  point P175 (142.4977, -39.7039)
  point P176 (145.1002, -40.1891)
  point P177 (147.6068, -40.6554)
  point P178 (150.0151, -41.1024)
  point P179 (152.3223, -41.5297)
  point P180 (154.5263, -41.9372)
  point P181 (156.6247, -42.324)
  point P182 (158.6153, -42.6903)
  point P183 (160.4961, -43.0357)
  point P184 (162.265, -43.3597)
  point P185 (163.9203, -43.6624)
  point P186 (165.4603, -43.9435)
  point P187 (166.883, -44.2026)
  point P188 (168.1872, -44.4397)
  point P189 (169.3715, -44.6545)
  point P190 (170.4343, -44.8473)
  point P191 (171.375, -45.0174)
  point P192 (172.1924, -45.1651)
  point P193 (172.8852, -45.2902)
  point P194 (173.4535, -45.3926)
  point P195 (173.8959, -45.4725)
  point P196 (174.2123, -45.5293)
  point P197 (174.4022, -45.5635)
  point P198 (-25.9, 8)
  point P199 (-51.52, 18)
  dimension "d21" = 10.3
  dimension "d22" = 77.28
  dimension "d100" = 10.2
  dimension "d101" = 4.2
  dimension "d103" = 10.2
  dimension "d104" = 4.2
  dimension "d164" = 25.9
  dimension "d165" = 8
  dimension "d167" = 51.52
  dimension "d168" = 18
  dimension "d267" = 10.2
  dimension "d268" = 4.2
  dimension "d269" = 44.25
  dimension "d270" = 7
  dimension "d271" = 10.2
  dimension "d272" = 4.2
  dimension "d273" = 70
  dimension "d274" = 17
  constraints: 48 end point, 8 midpoint, 8 parallel, 4 horizontal, 4 perpendicular, 1 centre point, 201 other
  measures "d21" diameter of A0
  measures "d22" distance of A0.centre point (-74.771, 19.532)
  measures "d100" distance of L2.end L1.end
  measures "d101" distance of L1.end L0.end
  measures "d103" distance of L8.end L7.end
  measures "d104" distance of L7.end L6.end
  measures "d164" horizontal distance of point (0, 0) point (-25.9, 8)
  measures "d165" vertical distance of point (0, 0) point (-25.9, 8)
  measures "d167" horizontal distance of point (0, 0) point (-51.52, 18)
  measures "d168" vertical distance of point (0, 0) point (-51.52, 18)
  measures "d267" distance of L14.end L13.end
  measures "d268" distance of L13.end L12.end
  measures "d269" horizontal distance of point (0, 0) point (44.25, -7)
  measures "d270" vertical distance of point (0, 0) point (44.25, -7)
  measures "d271" distance of L19.end L20.end
  measures "d272" distance of L18.end L19.end
  measures "d273" horizontal distance of point (0, 0) point (70, -17)
  measures "d274" vertical distance of point (0, 0) point (70, -17)